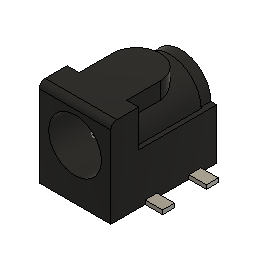
BarrelJackSMD v3 (Autodesk Fusion 360 design; units mm, degrees)
Autodesk Fusion 360 part; units mm, degrees
note: some values were not read from the file. Chosen so that the rebuilt part matches the saved one: which face or edge a step refers to. Set by a fixed rule: which sketch regions a step uses.
sketch "Sketch1" plane through (0, 0, 0) normal (0, 1, 0) x (1, 0, 0)
  line L0 (4.5, -6.65) -> (-4.5, -6.65)
  line L1 (-4.5, -6.65) -> (-4.5, 6.65)
  line L2 (-4.5, 6.65) -> (4.5, 6.65)
  line L3 (4.5, 6.65) -> (4.5, -6.65)
  line L4 (4.5, -6.65) -> (-4.5, 6.65) construction
  line L5 (-4.5, -6.65) -> (4.5, 6.65) construction
  line L6 (4.5, -6.65) -> (1.65, -6.65)
  line L7 (1.65, -6.65) -> (1.65, 8.05)
  line L8 (1.65, 8.05) -> (4.5, 8.05)
  line L9 (4.5, 8.05) -> (4.5, -6.65)
  line L10 (-3, -6.65) -> (3, -6.65)
  line L11 (3, -6.65) -> (3, 1.05)
  line L12 (-3, 1.05) -> (-3, -6.65)
  line L13 (0, 0) -> (0, 4.05) construction
  arc A0 (3, 1.05) -> (-3, 1.05) centre (0, 1.05) ccw
  line L14 (4.5, -6.65) -> (-4.5, -6.65)
  line L15 (-4.5, -6.65) -> (-4.5, -3.15)
  line L16 (-4.5, -3.15) -> (4.5, -3.15)
  line L17 (4.5, -3.15) -> (4.5, -6.65)
  line L18 (-6.7, -0.85) -> (6.7, -0.85)
  line L19 (6.7, -0.85) -> (6.7, -2.35)
  line L20 (6.7, -2.35) -> (-6.7, -2.35)
  line L21 (-6.7, -2.35) -> (-6.7, -0.85)
  line L22 (-6.7, 4.65) -> (6.7, 4.65)
  line L23 (6.7, 4.65) -> (6.7, 3.15)
  line L24 (6.7, 3.15) -> (-6.7, 3.15)
  line L25 (-6.7, 3.15) -> (-6.7, 4.65)
  circle A1 centre (0, -1.65) radius 0.675
  circle A2 centre (0, 2.65) radius 0.675
  dimension "d1" = 9
  dimension "d2" = 13.3
  dimension "d3" = 2.85
  dimension "d4" = 14.7
  dimension "d5" = 6
  dimension "d7" = 6
  dimension "d8" = 10.7
  dimension "d9" = 9
  dimension "d10" = 3.5
  dimension "d11" = 1.5
  dimension "d12" = 1.5
  dimension "d13" = 4.3
  dimension "d14" = 9.8
  dimension "d15" = 2.2
  dimension "d16" = 2.2
  dimension "d25" = 5
  dimension "d26" = 9.3
  dimension "d27" = 1.35
  dimension "d28" = 1.35
  measures "d7" diameter of A0
  measures "d8" distance of L10
  measures "d13" distance of L14 L20
  measures "d14" distance of L6 L24
  measures "d15" distance of L3 L23
  measures "d16" distance of L1
  measures "d25" distance of L0
  measures "d26" distance of L0
  measures "d27" diameter of A1
  measures "d28" diameter of A2
extrude "Extrude1" add sketch "Sketch1" along normal blind 6.35 contours L0 L3 L6 L9 L11 L14 L16 L17 | L0 L6 L7 L10 L11 L14 L16 | L3 L9 L11 L16 L20 | L0 L7 L10 L12 L14 L16 | L7 L11 L16 L20 | L3 L9 L11 L18 L20 | L0 L1 L12 L14 L15 L16 | L7 L12 L16 L20 | L7 L11 L18 L20 | L3 L9 L11 A0 L18 L24 | L1 L12 L16 L20 | L7 L12 L18 L20 | L7 L11 A0 L18 L24 | L3 L7 L9 A0 L22 L24 | L1 L12 L18 L20 | L7 L12 A0 L18 L24 A2 | L2 L3 L7 L9 L22 | L7 A0 L24 | L1 L12 A0 L18 L24 | L7 A0 L24 A2 | L1 L2 L7 L22 | L1 L7 A0 L22 L24 | L24 A2 | L24 A2 | A1 makes body 1
sketch "Sketch2" plane through (0, 6.35, 0) normal (0, 1, 0) x (-1, 0, 0)
  line L0 (-4.5, 6.65) -> (-4.5, -6.65)
  line L1 (-4.5, -6.65) -> (4.5, -6.65)
  line L2 (4.5, -6.65) -> (4.5, 6.65)
  line L3 (4.5, 6.65) -> (-4.5, 6.65)
  line L4 (3.93, 6.65) -> (-3.93, 6.65)
  line L5 (-3.93, 6.65) -> (-3.93, -5.25)
  line L6 (-3.93, -5.25) -> (3.93, -5.25)
  line L7 (3.93, -5.25) -> (3.93, 6.65)
  line L8 (3.7499, 6.65) -> (-3.7499, 6.65)
  line L9 (-3.7499, 6.65) -> (-3.7499, -6.65)
  line L10 (-3.7499, -6.65) -> (3.7499, -6.65)
  line L11 (3.7499, -6.65) -> (3.7499, 6.65)
  line L12 (6.7, -4.65) -> (-6.7, -4.65)
  line L13 (0, 0) -> (0, -4.3382) construction
  line L14 (0, -6.65) -> (0, 6.65)
  dimension "d19" = 7.86
  dimension "d20" = 11.9
revolve "Revolve1" add sketch "Sketch2" angle 360 about axis through (0, 6.35, -6.65) along (0, 0, 1) contours L3 L4 L8 L11 L12 L14 | L6 L11 L12 L14 | L3 L4 L7 L11 L12 | L6 L7 L11 L12 bodies 1
extrude "Extrude2" add sketch "Sketch1" along normal blind 11 contours L0 L3 L6 L9 L11 L14 L16 L17 | L0 L6 L7 L10 L11 L14 L16 | L0 L7 L10 L12 L14 L16 | L7 L11 L16 L20 | L0 L1 L12 L14 L15 L16 | L7 L12 L16 L20 | L7 L11 L18 L20 | L7 L12 L18 L20 | L7 L11 A0 L18 L24 | L7 L12 A0 L18 L24 A2 | L7 A0 L24 | L7 A0 L24 A2 | L24 A2 | L24 A2 | A1 bodies 1
revolve "Revolve2" add sketch "Sketch2" angle 360 about axis through (0, 6.35, -6.65) along (0, 0, 1) contours L1 L6 L10 L11 L14 bodies 1
extrude "Extrude3" add sketch "Sketch1" against normal blind 1.2 contours L24 A2 | L24 A2 | A1 bodies 1
chamfer "Chamfer1" distance 0.3 angle 45 2 edges at (-0.6293, -1.2, 1.4059) (-0.6293, -1.2, -2.8941) on bodies 1
extrude "Extrude4" add sketch "Sketch1" along normal blind 0.5 contours L3 L9 L18 L19 L20 | L3 L9 L22 L23 L24 | L1 L18 L20 L21 | L1 L22 L24 L25 bodies 1
sketch "Sketch3" plane through (0, 0, -6.65) normal (0, 0, -1) x (-1, 0, 0)
  line L0 (-3.7499, 6.35) -> (-4.5, 6.35)
  line L1 (-4.5, 6.35) -> (-4.5, 0)
  line L2 (-4.5, 0) -> (4.5, 0)
  line L3 (4.5, 0) -> (4.5, 6.35)
  line L4 (4.5, 6.35) -> (3.7499, 6.35)
  arc A0 (3.7499, 6.35) -> (-3.7499, 6.35) centre (0, 6.35) ccw
  circle A1 centre (0, 6.35) radius 3.3
  circle A2 centre (0, 6.35) radius 0.8
  dimension "d34" = 6.6
  dimension "d38" = 1.6
  measures "d34" diameter of A1
  measures "d38" diameter of A2
extrude "Extrude5" cut sketch "Sketch3" along normal blind 12 from surface at -13.3 contours A1 | A2 bodies 1
extrude "Extrude6" add sketch "Sketch3" against normal blind 11 contours A2 bodies 1
fillet "Fillet1" radius 0.75 1 edges at (0.7459, 6.6393, 4.35) on bodies 1
fillet "Fillet2" radius 0.75 1 edges at (0, 11, 6.65) on bodies 1
copy_body "Body->Comp1" bodies 1 removing the originals makes body 2 in component "BarrelJack"
component "BarrelJack" placed x (1, 0, 0) y (0, 1, 0) z (0, 0, 1) at (0, 0, 0)
